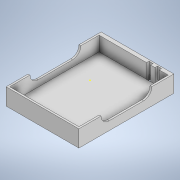
# Autodesk Inventor part: battery-cover
Saved by Autodesk Inventor 2021.2 (Build 252289000, 289)
## iProperties
Created: 2021-04-01
Part Number: battery-cover
Material: Generic
Document SubType Name: Modeling
Designer: Nick
Density: 1 g/cm^3
Appearance: Default
Author: Nick
Autodesk Inventor part; units mm, degrees
ref_plane "YZ Plane" through (0, 0, 0) normal (1, 0, 0) x (0, 1, 0)
ref_plane "XZ Plane" through (0, 0, 0) normal (0, 1, 0) x (-1, 0, 0)
ref_plane "XY Plane" through (0, 0, 0) normal (0, 0, 1) x (1, 0, 0)
sketch "Sketch1" plane through (0, 0, 0) normal (0, 1, 0) x (-1, 0, 0)
  line L0 (17.9, -23.35) -> (-17.9, -23.35)
  line L1 (-17.9, -23.35) -> (-17.9, 23.35)
  line L2 (-17.9, 23.35) -> (17.9, 23.35)
  line L3 (17.9, 23.35) -> (17.9, -23.35)
  point P0 (0, 0)
  dimension "d0" = 35.8
  dimension "d1" = 46.7
  dimension "d2" = 23.35
  dimension "d3" = 17.9
  constraints: 8 end point, 2 parallel, 1 horizontal, 1 perpendicular
  measures "d0" distance of L1.end L2.end
  measures "d1" distance of L2.end L0.start
  measures "d2" distance from line of point (0, 0) L0
  measures "d3" distance from line of point (0, 0) L1
extrude "Extrusion1" add sketch "Sketch1" along normal blind 8.2
sketch "Sketch2" plane through (0, 8.2, 0) normal (0, 1, 0) x (1, 0, 0)
  line L0 (-16.8, -22.25) -> (16.8, -22.25)
  line L1 (16.8, -22.25) -> (16.8, 21.35)
  line L2 (16.8, 21.35) -> (-16.8, 21.35)
  line L3 (-16.8, 21.35) -> (-16.8, -22.25)
  line L4 (-17.9, -23.35) -> (17.9, -23.35) projected
  line L5 (17.9, -23.35) -> (17.9, 23.35) projected
  line L6 (-17.9, 23.35) -> (-17.9, -23.35) projected
  line L7 (17.9, 23.35) -> (-17.9, 23.35) projected
  point P0 (0, 0)
  dimension "d6" = 1.1
  dimension "d7" = 1.1
  dimension "d8" = 1.1
  dimension "d9" = 2
  constraints: 8 end point, 2 parallel, 1 horizontal, 1 perpendicular
  measures "d6" distance between parallel lines of L0 L4
  measures "d7" distance between parallel lines of L5 L1
  measures "d8" distance between parallel lines of L6 L3
  measures "d9" distance between parallel lines of L7 L2
extrude "Extrusion2" cut sketch "Sketch2" against normal blind 7.1 contours L3 L2 L1 L0
sketch "Sketch6" plane through (17.9, 0, 23.35) normal (1, 0, 0) x (0, 0, -1)
  line L0 (1.1, 8.2) -> (44.7, 8.2) projected
  line L1 (10.85, 8.2) -> (35.85, 8.2)
  line L2 (35.85, 8.2) -> (35.85, 4.2)
  line L3 (35.85, 4.2) -> (10.85, 4.2)
  line L4 (10.85, 4.2) -> (10.85, 8.2)
  line L5 (46.7, 0) -> (46.7, 8.2) projected
  point P0 (23.35, 0)
  dimension "d34" = 25
  dimension "d35" = 10.85
  dimension "d36" = 4
  constraints: 8 end point, 2 parallel, 1 horizontal, 1 perpendicular, 1 point on line
  measures "d34" distance of L2.end L3.end
  measures "d35" distance between parallel lines of L5 L2
  measures "d36" distance of L1.end L2.end
extrude "Extrusion6" cut sketch "Sketch6" against normal through all
fillet "Fillet2" radius 4 4 edges at (17.35, 4.2, 12.5) (-17.35, 4.2, 12.5) (-17.35, 4.2, -12.5) (17.35, 4.2, -12.5)
sketch "Sketch9" plane through (0, 8.2, 0) normal (0, 1, 0) x (1, 0, 0)
  point P0 (0, 0)
sketch "Sketch10" plane through (0, 8.2, 0) normal (0, 1, 0) x (1, 0, 0)
  line L0 (-16.8, 21.35) -> (16.8, 21.35) projected
  line L1 (12.55, 21.35) -> (10.55, 21.35)
  line L2 (10.55, 21.35) -> (10.55, 22.35)
  line L3 (10.55, 22.35) -> (12.55, 22.35)
  line L4 (12.55, 22.35) -> (12.55, 21.35)
  line L5 (8.345, 21.35) -> (6.345, 21.35)
  line L6 (6.345, 21.35) -> (6.345, 22.35)
  line L7 (6.345, 22.35) -> (8.345, 22.35)
  line L8 (8.345, 22.35) -> (8.345, 21.35)
  line L9 (17.9, 23.35) -> (-17.9, 23.35) projected
  line L10 (17.9, 12.5) -> (17.9, 23.35) projected
  point P0 (0, 0)
  dimension "d51" = 2
  dimension "d52" = 2
  dimension "d53" = 2.205
  dimension "d54" = 1
  dimension "d55" = 5.35
  constraints: 16 end point, 4 parallel, 3 point on line, 2 horizontal, 2 perpendicular
  measures "d51" distance of L2.end L3.end
  measures "d52" distance of L6.end L7.end
  measures "d53" distance between parallel lines of L8 L2
  measures "d54" distance between parallel lines of L9 L7
  measures "d55" distance between parallel lines of L10 L4
extrude "Extrusion9" cut sketch "Sketch10" against normal through all
sketch "Sketch11" plane through (0, 8.2, 0) normal (0, 1, 0) x (1, 0, 0)
  line L0 (-17, 21.45) -> (17, 21.45)
  line L1 (17, 21.45) -> (17, -22.45)
  line L2 (17, -22.45) -> (-17, -22.45)
  line L3 (-17, -22.45) -> (-17, 21.45)
  line L4 (16.8, -22.25) -> (-16.8, -22.25) projected
  line L5 (16.8, -12.5) -> (16.8, -22.25) projected
  line L6 (-16.8, 21.35) -> (6.345, 21.35) projected
  line L7 (-16.8, 12.5) -> (-16.8, 21.35) projected
  point P0 (0, 0)
  dimension "d58" = 0.2
  dimension "d59" = 0.2
  dimension "d60" = 0.1
  dimension "d61" = 0.2
  constraints: 8 end point, 2 parallel, 1 horizontal, 1 perpendicular
  measures "d58" distance between parallel lines of L4 L2
  measures "d59" distance between parallel lines of L5 L1
  measures "d60" distance between parallel lines of L0 L6
  measures "d61" distance between parallel lines of L7 L3
extrude "Extrusion10" cut sketch "Sketch11" against normal up to surface (7.1 mm away)
sketch "Sketch12" plane through (0, 8.2, 0) normal (0, 1, 0) x (1, 0, 0)
  line L0 (6.345, 22.35) -> (8.345, 22.35) projected
  line L1 (6.345, 22.35) -> (8.345, 22.35)
  line L2 (8.345, 22.35) -> (8.345, 22.649)
  line L3 (8.345, 22.649) -> (6.345, 22.649)
  line L4 (6.345, 22.649) -> (6.345, 22.35)
  line L5 (10.55, 22.35) -> (12.55, 22.35) projected
  line L6 (10.55, 22.35) -> (12.5613, 22.35)
  line L7 (12.5613, 22.35) -> (12.5613, 22.649)
  line L8 (12.5613, 22.649) -> (10.55, 22.649)
  line L9 (10.55, 22.649) -> (10.55, 22.35)
  point P0 (0, 0)
  constraints: 16 end point, 4 parallel, 2 horizontal, 2 perpendicular, 1 point on line
extrude "Extrusion11" cut sketch "Sketch12" against normal through all
sketch "Sketch13" plane through (17.9, 0, -23.35) normal (0, 0, -1) x (-1, 0, 0)
  line L0 (7.35, 0) -> (5.35, 0) projected
  line L1 (7.35, 8.2) -> (7.35, 1.1) projected
  line L2 (5.35, 0) -> (7.35, 0)
  line L3 (7.35, 0) -> (7.35, 2.5)
  line L4 (7.35, 2.5) -> (5.35, 2.5)
  line L5 (5.35, 2.5) -> (5.35, 0)
  line L6 (11.555, 0) -> (9.555, 0) projected
  line L7 (11.555, 8.2) -> (11.555, 1.1) projected
  line L8 (9.555, 0) -> (11.555, 0)
  line L9 (11.555, 0) -> (11.555, 2.5)
  line L10 (11.555, 2.5) -> (9.555, 2.5)
  line L11 (9.555, 2.5) -> (9.555, 0)
  point P0 (17.9, 0)
  dimension "d66" = 2.5
  constraints: 16 end point, 4 parallel, 3 point on line, 2 horizontal, 2 perpendicular
  measures "d66" distance of L4.end L0.end
extrude "Extrusion12" cut sketch "Sketch13" against normal up to surface (2 mm away)
body "Solid1"
